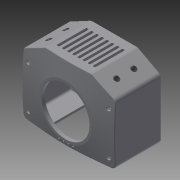
# Autodesk Inventor part: Enclosure01
Saved by Autodesk Inventor 2013 (Build 170138000, 138)
## iProperties
Created: 2014-04-13
Part Number: Enclosure01
Material: Generic
Document SubType Name: Modeling
Designer: spichelh
Density: 1 g/cm^3
Author: spichelh
Autodesk Inventor part; units mm, degrees
ref_plane "YZ Plane" through (0, 0, 0) normal (1, 0, 0) x (0, 1, 0)
ref_plane "XZ Plane" through (0, 0, 0) normal (0, 1, 0) x (-1, 0, 0)
ref_plane "XY Plane" through (0, 0, 0) normal (0, 0, 1) x (1, 0, 0)
sketch "Sketch1" plane through (0, 0, 0) normal (0, 0, 1) x (1, 0, 0)
  circle A0 centre (31.4469, 31.0185) radius 28
  line L0 (-19.3531, 19.423) -> (82.2469, 19.423) construction
  line L1 (7.9639, 76.573) -> (-19.3531, 76.573) construction
  line L2 (82.2469, 76.573) -> (53.8439, 76.573) construction
  line L3 (82.2469, 19.423) -> (82.2469, 76.573) construction
  line L4 (-19.3531, 76.573) -> (-19.3531, 19.423) construction
  line L5 (5.509, 60.2207) -> (61.389, 60.2207) construction
  line L6 (61.389, 60.2207) -> (61.389, 72.2207) construction
  line L7 (61.389, 72.2207) -> (5.509, 72.2207) construction
  line L8 (5.509, 72.2207) -> (5.509, 60.2207) construction
  circle A1 centre (61.389, 6.2635) radius 1.5 construction
  circle A2 centre (61.389, 55.7935) radius 1.5 construction
  circle A3 centre (5.509, 55.7935) radius 1.5 construction
  circle A4 centre (5.0259, 23.233) radius 1.5 construction
  arc A5 (5.509, 7.6907) -> (5.509, 1.6907) centre (5.509, 4.6907) ccw construction
  line L9 (5.509, 1.6907) -> (5.509, -3.7465) construction
  line L10 (5.509, -3.7465) -> (61.389, -3.7465) construction
  line L11 (61.389, -3.7465) -> (61.389, 1.6907) construction
  arc A6 (61.389, 1.6907) -> (61.389, 7.6907) centre (61.389, 4.6907) ccw construction
  line L12 (61.389, 7.6907) -> (61.389, 51.2207) construction
  arc A7 (61.389, 51.2207) -> (61.389, 57.2207) centre (61.389, 54.2207) ccw construction
  line L13 (61.389, 57.2207) -> (61.389, 60.2207) construction
  line L14 (61.389, 60.2207) -> (5.509, 60.2207) construction
  line L15 (5.509, 60.2207) -> (5.509, 57.2207) construction
  arc A8 (5.509, 57.2207) -> (5.509, 51.2207) centre (5.509, 54.2207) ccw construction
  line L16 (5.509, 51.2207) -> (5.509, 7.6907) construction
  line L17 (-22.3531, -3.7465) -> (85.2469, -3.7465)
  line L18 (85.2469, -3.7465) -> (85.2469, 66.2535)
  line L19 (58.3159, 80.573) -> (4.578, 80.573)
  line L20 (31.4469, -3.7465) -> (31.4469, 78.2535) construction
  circle A9 centre (31.4469, 31.0185) radius 23 projected
  line L21 (-22.3531, 66.2535) -> (4.578, 80.573)
  line L22 (-22.3531, 66.2535) -> (-22.3531, -3.7465)
  line L23 (85.2469, 66.2535) -> (58.3159, 80.573)
  point P0 (0, 0)
  dimension "d42" = 0
  dimension "d44" = 3
  dimension "d45" = 4
  dimension "d46" = 4
  dimension "d47" = 57.15
  dimension "d48" = 57.15
  dimension "d49" = 101.6
  dimension "d50" = 3.81
  dimension "d59" = 56
  dimension "d199" = 70
  dimension "d200" = 118
  dimension "d201" = 84.3195
  dimension "d202" = 107.6
  constraints: 48 end point, 9 centre point, 8 point on circle, 2 parallel, 2 symmetric about line, 1 concentric, 1 horizontal, 1 midpoint, 1 perpendicular, 1 point on line
  measures "d42" distance between parallel lines of L17 L10
  measures "d44" distance between parallel lines of L18 L3
  measures "d45" distance between parallel lines of L19 L1
  measures "d46" distance between parallel lines of L19 L2
  measures "d47" distance between parallel lines of L0 L1
  measures "d48" distance between parallel lines of L2 L0
  measures "d49" distance between parallel lines of L4 L3
  measures "d50" distance from line of L0 A4.centre
  measures "d59" diameter of A0
  measures "d199" distance of L21.start L17.start
  measures "d200" angle of L22 L21
  measures "d201" distance between parallel lines of L17 L19
  measures "d202" distance between parallel lines of L22 L18
extrude "Extrusion1" add sketch "Sketch1" along normal blind 11 contours L22 L21 L19 L23 L18 L17
sketch "Sketch4" plane through (0, 0, 11) normal (0, 0, 1) x (1, 0, 0)
  circle A0 centre (-15.5431, 55.7835) radius 1.5 projected
  circle A1 centre (-15.5431, 6.2535) radius 1.5 projected
  circle A2 centre (78.4369, 6.2535) radius 1.5 projected
  circle A3 centre (78.4369, 55.7835) radius 1.5 projected
  point P0 (0, 0)
extrude "Extrusion3" cut sketch "Sketch4" against normal blind 10
sketch "Sketch25" plane through (0, 0, 11) normal (0, 0, 1) x (1, 0, 0)
  circle A0 centre (31.4469, 31.019) radius 31
  circle A1 centre (31.4469, 31.019) radius 28
  line L0 (58.3159, 80.573) -> (4.578, 80.573) projected
  circle A2 centre (31.4469, 31.0185) radius 28 projected
  point P0 (0, 0)
  dimension "d196" = 62
  dimension "d198" = 49.554
  dimension "d203" = 0.0005
  constraints: 2 centre point, 1 coincident
  measures "d196" diameter of A0
  measures "d198" distance from line of L0 A0.centre
  measures "d203" distance of A0.centre A2.centre
extrude "Extrusion21" cut sketch "Sketch25" against normal blind 50 draft 82 contours A0 | A1 keep common part
sketch "Sketch2" plane through (0, 0, 0) normal (0, 0, -1) x (-1, 0, 0)
  circle A0 centre (-31.4469, 31.0185) radius 28 projected
  line L0 (22.3531, -3.7465) -> (-85.2469, -3.7465) projected
  line L1 (-58.3159, 80.573) -> (-4.578, 80.573) projected
  line L2 (-85.2469, -3.7465) -> (-85.2469, 66.2535) projected
  line L3 (-82.7469, 78.073) -> (19.8531, 78.073)
  line L4 (19.8531, 78.073) -> (19.8531, -1.2465)
  line L5 (19.8531, -1.2465) -> (-82.7469, -1.2465)
  line L6 (-82.7469, -1.2465) -> (-82.7469, 78.073)
  line L7 (22.3531, 66.2535) -> (22.3531, -3.7465) projected
  line L8 (-4.578, 80.573) -> (22.3531, 66.2535) projected
  line L9 (-85.2469, 66.2535) -> (-58.3159, 80.573) projected
  dimension "d51" = 2.5
  dimension "d52" = 2.5
  dimension "d54" = 2.5
  constraints: 8 end point, 2 parallel, 1 horizontal, 1 perpendicular
  measures "d51" distance between parallel lines of L3 L1
  measures "d52" distance between parallel lines of L2 L6
  measures "d54" distance between parallel lines of L0 L5
extrude "Extrusion2" add sketch "Sketch2" along normal blind 38 contours L0 L2 L9 L6 L5 L4 L8 L7 | L3 L9 L1 L8
ref_plane "Work Plane1" through (0, 0, 7) normal (0, 0, -1) x (-1, 0, 0)
sketch "Sketch28" plane through (0, 0, 7) normal (0, 0, -1) x (-1, 0, 0)
  circle A0 centre (-31.4469, 31.0185) radius 28 projected
  circle A1 centre (-31.4469, 31.0185) radius 31
  point P0 (0, 0)
  dimension "d209" = 62
  constraints: 1 centre point, 1 coincident
  measures "d209" diameter of A1
extrude "Extrusion23" cut sketch "Sketch28" along normal blind 50 draft 78 contours A0 | A1
sketch "Sketch5" plane through (-22.3531, 80.573, 10) normal (0, 1, 0) x (-1, 0, 0)
  line L0 (0, 0) -> (128.1647, 0)
  line L1 (36.0824, 63) -> (92.0824, 63)
  line L2 (92.0824, 63) -> (92.0824, 7)
  line L3 (92.0824, 7) -> (36.0824, 7)
  line L4 (36.0824, 7) -> (36.0824, 63)
  line L5 (64.0824, 0) -> (64.0824, -31.7336) construction
  line L6 (36.0824, 63) -> (92.0824, 7) construction
  line L7 (92.0824, 63) -> (36.0824, 7) construction
  line L8 (104.9242, 0) -> (-0.6758, 0)
  line L9 (87.1496, -1) -> (20.4504, -1) projected
  line L10 (-26.931, -48) -> (-80.669, -48) projected
  line L11 (16.7879, -48) -> (43.5691, -1) construction
  point P0 (19.351, -30)
  point P1 (64.0824, 35)
  point P2 (0, 48)
  point P3 (64.0824, 35)
  point P4 (20.4504, -1)
  dimension "d28" = 56
  dimension "d29" = 56
  dimension "d41" = 7
  constraints: 20 end point, 3 midpoint, 3 parallel, 2 point on line, 1 collinear, 1 horizontal, 1 perpendicular, 4 other
  measures "d28" distance of L2.end L3.end
  measures "d29" distance of L1.end L2.end
  measures "d41" distance between parallel lines of L8 L3
extrude "Extrusion4" cut sketch "Sketch5" against normal blind 100
sketch "Sketch6" plane through (-6.7798, 80.573, 3) normal (0, 1, 0) x (1, 0, 0)
  line L0 (71.5763, -7) -> (-25.8, -7) projected
  line L1 (0, 0) -> (56, 0)
  line L2 (56, 0) -> (56, -7)
  line L3 (56, -7) -> (0, -7)
  line L4 (0, -7) -> (0, 0)
  point P0 (76.8, -7)
  point P1 (-20.8, -7)
  point P2 (6.7798, 3)
  point P3 (71.5763, -8)
  point P4 (-25.8, -7)
  constraints: 8 end point, 2 parallel, 1 horizontal, 1 perpendicular, 2 other
extrude "Extrusion5" [suppressed]
fillet "Fillet9" radius 5 6 edges at (85.2469, -3.7465, 3.1642) (-22.3531, -3.7465, 3.1642) (-22.3531, 66.2535, 3.1189) (4.578, 80.573, 4.521) (58.3159, 80.573, 4.521) (85.2469, 66.2535, 3.1189)
sketch "Sketch24" plane through (31.4469, 31.0185, 3) normal (0, 0, -1) x (0.9394635, -0.3426491, 0)
  arc A0 (-28, 0) -> (28, 0) centre (0, 0) ccw projected
  circle A1 centre (0, 0) radius 28
  point P0 (-18.9148, 39.916)
  dimension "d186" = 56
  constraints: 1 centre point, 1 coincident
  measures "d186" diameter of A1
extrude "Extrusion20" [suppressed]
ref_plane "Work Plane2" through (0, 0, 6) normal (0, 0, 1) x (1, 0, 0)
sketch "Sketch7" plane through (0, 0, 11) normal (0, 0, 1) x (1, 0, 0)
  line L0 (-22.3531, -3.7465) -> (85.2469, -3.7465) projected
  line L1 (59.4469, 75.7535) -> (3.4469, 75.7535) projected
  line L2 (31.4469, -3.7465) -> (31.4469, 75.7535) construction
  line L3 (23.1969, -0.7465) -> (23.1969, -0.7465)
  line L4 (22.1969, 0.2535) -> (22.1969, 1.2535)
  line L5 (23.1969, 2.2535) -> (23.1969, 2.2535)
  line L6 (24.1969, 1.2535) -> (24.1969, 0.2535)
  arc A0 (24.1969, 1.2535) -> (23.1969, 2.2535) centre (23.1969, 1.2535) ccw
  arc A1 (23.1969, 2.2535) -> (22.1969, 1.2535) centre (23.1969, 1.2535) ccw
  arc A2 (22.1969, 0.2535) -> (23.1969, -0.7465) centre (23.1969, 0.2535) ccw
  arc A3 (23.1969, -0.7465) -> (24.1969, 0.2535) centre (23.1969, 0.2535) ccw
  line L7 (27.6969, 0.2535) -> (27.6969, 1.2535)
  line L8 (29.6969, 1.2535) -> (29.6969, 0.2535)
  arc A4 (29.6969, 1.2535) -> (28.6969, 2.2535) centre (28.6969, 1.2535) ccw
  arc A5 (28.6969, 2.2535) -> (27.6969, 1.2535) centre (28.6969, 1.2535) ccw
  arc A6 (27.6969, 0.2535) -> (28.6969, -0.7465) centre (28.6969, 0.2535) ccw
  arc A7 (28.6969, -0.7465) -> (29.6969, 0.2535) centre (28.6969, 0.2535) ccw
  line L9 (33.1969, 0.2535) -> (33.1969, 1.2535)
  line L10 (35.1969, 1.2535) -> (35.1969, 0.2535)
  arc A8 (35.1969, 1.2535) -> (34.1969, 2.2535) centre (34.1969, 1.2535) ccw
  arc A9 (34.1969, 2.2535) -> (33.1969, 1.2535) centre (34.1969, 1.2535) ccw
  arc A10 (33.1969, 0.2535) -> (34.1969, -0.7465) centre (34.1969, 0.2535) ccw
  arc A11 (34.1969, -0.7465) -> (35.1969, 0.2535) centre (34.1969, 0.2535) ccw
  line L11 (38.6969, 0.2535) -> (38.6969, 1.2535)
  line L12 (40.6969, 1.2535) -> (40.6969, 0.2535)
  arc A12 (40.6969, 1.2535) -> (39.6969, 2.2535) centre (39.6969, 1.2535) ccw
  arc A13 (39.6969, 2.2535) -> (38.6969, 1.2535) centre (39.6969, 1.2535) ccw
  arc A14 (38.6969, 0.2535) -> (39.6969, -0.7465) centre (39.6969, 0.2535) ccw
  arc A15 (39.6969, -0.7465) -> (40.6969, 0.2535) centre (39.6969, 0.2535) ccw
  line L13 (29.6969, 0.7535) -> (33.1969, 0.7535) construction
  point P0 (-17.3531, -3.7465)
  point P1 (80.2469, -3.7465)
  point P2 (0, 0)
  point P3 (24.1969, -0.7465)
  point P4 (22.1969, 2.2535)
  point P5 (24.1969, 2.2535)
  point P6 (29.6969, -0.7465)
  point P7 (27.6969, 2.2535)
  point P8 (29.6969, 2.2535)
  point P9 (35.1969, -0.7465)
  point P10 (33.1969, 2.2535)
  point P11 (35.1969, 2.2535)
  point P12 (40.6969, -0.7465)
  point P13 (38.6969, 2.2535)
  point P14 (40.6969, 2.2535)
  point P15 (31.4469, 0.7535)
  dimension "d64" = 2
  dimension "d66" = 3
  dimension "d67" = 1
  dimension "d68" = 1
  dimension "d69" = 4
  dimension "d78" = 16.5
  dimension "d79" = 7.25
  dimension "d80" = 7.25
  constraints: 32 point on circle, 24 end point, 16 centre point, 16 point on line, 8 tangent, 5 midpoint, 2 equal radius, 2 parallel, 1 horizontal, 1 perpendicular
  measures "d64" distance of point (22.197, 2.253) point (24.197, 2.253)
  measures "d66" distance of point (24.197, 2.253) point (24.197, -0.747)
  measures "d67" radius of A0
  measures "d68" radius of A3
  measures "d69" distance from line of L0 A3.centre
  measures "d78" distance of A14.centre A3.centre
  measures "d79" distance from line of L6 point (31.447, 0.753)
  measures "d80" distance from line of point (31.447, 0.753) L11
extrude "Extrusion6" cut sketch "Sketch7" against normal blind 5
sketch "Sketch31" plane through (0, 0, 6) normal (0, 0, 1) x (1, 0, 0)
  line L0 (85.2469, 1.2535) -> (85.2469, 63.2492) projected
  line L1 (82.5943, 67.6639) -> (59.4166, 79.9877) projected
  line L2 (57.0693, 80.573) -> (5.8246, 80.573) projected
  line L3 (3.4773, 79.9877) -> (-19.7004, 67.6639) projected
  line L4 (-22.3531, 63.2492) -> (-22.3531, 1.2535) projected
  line L5 (-17.3531, -3.7465) -> (80.2469, -3.7465) projected
  arc A0 (29.6799, 0.0694) -> (33.214, 0.0694) centre (31.4469, 31.019) ccw projected
  arc A1 (24.1969, 0.8787) -> (27.697, 0.2466) centre (31.4469, 31.019) ccw projected
  line L6 (24.1969, 0.8787) -> (24.1969, 0.2535) projected
  line L7 (22.1969, 0.2535) -> (22.1969, 1.2535) projected
  arc A2 (40.6819, 1.4265) -> (22.212, 1.4265) centre (31.4469, 31.019) ccw projected
  line L8 (40.6969, 1.2535) -> (40.6969, 0.2535) projected
  line L9 (38.6969, 0.2535) -> (38.6969, 0.8787) projected
  arc A3 (35.1969, 0.2466) -> (38.6969, 0.8787) centre (31.4469, 31.019) ccw projected
  spline S0 degree 5 poles (79.9369, 6.2535) (79.9369, 6.4896) (79.8901, 6.7131) (79.8078, 6.9142) (79.6985, 7.089) (79.3892, 7.444) (79.1712, 7.6007) (78.9248, 7.7086) (78.6593, 7.7625) (78.197, 7.7457) (78.0071, 7.7107) (77.815, 7.6419) (77.6284, 7.5361) (77.2941, 7.2495) (77.1462, 7.0707) (77.0327, 6.8552) (76.9691, 6.6321) (76.9219, 6.1944) (76.9403, 5.9806) (76.9923, 5.7833) (77.0708, 5.6069) (77.3344, 5.1912) (77.5564, 4.9876) (77.8147, 4.8424) (78.1045, 4.759) (78.6051, 4.7503) (78.8055, 4.7777) (79.0097, 4.8419) (79.2089, 4.9467) (79.5873, 5.2569) (79.7624, 5.4705) (79.8851, 5.7352) (79.9369, 6.0009) (79.9369, 6.2535) knots 0 0 0 0 0 0 0.115502 0.115502 0.115502 0.115502 0.273569 0.273569 0.273569 0.273569 0.379516 0.379516 0.379516 0.379516 0.484537 0.484537 0.484537 0.484537 0.590505 0.590505 0.590505 0.590505 0.765499 0.765499 0.765499 0.765499 0.876442 0.876442 0.876442 0.876442 1 1 1 1 1 1 projected
  spline S1 degree 5 poles (-14.0431, 55.7835) (-14.0431, 56.0034) (-14.0836, 56.2117) (-14.1553, 56.401) (-14.2511, 56.5681) (-14.5342, 56.9259) (-14.7425, 57.0919) (-14.9815, 57.2113) (-15.2422, 57.2785) (-15.7112, 57.2866) (-15.9117, 57.2593) (-16.1159, 57.1951) (-16.3151, 57.0902) (-16.6735, 56.7964) (-16.8328, 56.6087) (-16.9533, 56.3798) (-17.0179, 56.1423) (-17.0573, 55.6805) (-17.031, 55.457) (-16.9684, 55.2523) (-16.8776, 55.0716) (-16.5871, 54.6638) (-16.3545, 54.472) (-16.0886, 54.3411) (-15.7951, 54.2733) (-15.3031, 54.2912) (-15.1133, 54.3263) (-14.9212, 54.3951) (-14.7345, 54.5009) (-14.3755, 54.8087) (-14.208, 55.0203) (-14.0917, 55.2804) (-14.0431, 55.5385) (-14.0431, 55.7835) knots 0 0 0 0 0 0 0.108338 0.108338 0.108338 0.108338 0.265313 0.265313 0.265313 0.265313 0.376257 0.376257 0.376257 0.376257 0.487434 0.487434 0.487434 0.487434 0.598396 0.598396 0.598396 0.598396 0.773389 0.773389 0.773389 0.773389 0.879335 0.879335 0.879335 0.879335 1 1 1 1 1 1 projected
  spline S2 degree 5 poles (-14.0431, 6.2535) (-14.0431, 6.4984) (-14.0918, 6.7565) (-14.208, 7.0166) (-14.3755, 7.2282) (-14.7345, 7.5361) (-14.9212, 7.6419) (-15.1133, 7.7107) (-15.3031, 7.7457) (-15.7951, 7.7636) (-16.0886, 7.6958) (-16.3545, 7.5649) (-16.5871, 7.3732) (-16.8776, 6.9654) (-16.9684, 6.7847) (-17.031, 6.58) (-17.0573, 6.3564) (-17.0179, 5.8947) (-16.9533, 5.6571) (-16.8328, 5.4282) (-16.6735, 5.2406) (-16.3151, 4.9467) (-16.1159, 4.8419) (-15.9117, 4.7777) (-15.7112, 4.7503) (-15.2403, 4.7585) (-14.9778, 4.8266) (-14.7375, 4.9476) (-14.5284, 5.1157) (-14.2473, 5.4757) (-14.1531, 5.6418) (-14.0828, 5.8295) (-14.0431, 6.0358) (-14.0431, 6.2535) knots 0 0 0 0 0 0 0.120665 0.120665 0.120665 0.120665 0.226611 0.226611 0.226611 0.226611 0.401603 0.401603 0.401603 0.401603 0.512565 0.512565 0.512565 0.512565 0.623742 0.623742 0.623742 0.623742 0.734686 0.734686 0.734686 0.734686 0.892762 0.892762 0.892762 0.892762 1 1 1 1 1 1 projected
  spline S3 degree 5 poles (79.9369, 55.7835) (79.9369, 56.036) (79.885, 56.3017) (79.7624, 56.5664) (79.5873, 56.78) (79.2089, 57.0902) (79.0097, 57.1951) (78.8055, 57.2593) (78.6051, 57.2866) (78.1045, 57.2779) (77.8147, 57.1946) (77.5564, 57.0494) (77.3344, 56.8457) (77.0708, 56.43) (76.9923, 56.2537) (76.9403, 56.0564) (76.9219, 55.8426) (76.9691, 55.4049) (77.0327, 55.1817) (77.1462, 54.9663) (77.2941, 54.7875) (77.6284, 54.5009) (77.815, 54.3951) (78.0071, 54.3263) (78.197, 54.2912) (78.6612, 54.2743) (78.9285, 54.3291) (79.1763, 54.4385) (79.3953, 54.5974) (79.7026, 54.9547) (79.8101, 55.1285) (79.891, 55.3281) (79.9369, 55.5496) (79.9369, 55.7835) knots 0 0 0 0 0 0 0.123558 0.123558 0.123558 0.123558 0.234501 0.234501 0.234501 0.234501 0.409495 0.409495 0.409495 0.409495 0.515462 0.515462 0.515462 0.515462 0.620483 0.620483 0.620483 0.620483 0.726431 0.726431 0.726431 0.726431 0.885598 0.885598 0.885598 0.885598 1 1 1 1 1 1 projected
  line L10 (-14.4969, 56.8585) -> (-16.5892, 54.7085) construction
  line L11 (-16.618, 56.8296) -> (-14.4681, 54.7373) construction
  circle A4 centre (-15.5431, 55.7835) radius 2.5
  line L12 (31.4469, 31.019) -> (31.4469, 90.1404) construction
  circle A5 centre (78.4369, 55.7835) radius 2.5
  line L13 (31.4469, 31.019) -> (51.7757, 31.019) construction
  circle A6 centre (-15.5431, 6.2545) radius 2.5
  circle A7 centre (78.4369, 6.2545) radius 2.5
  point P0 (0, 0)
  dimension "d214" = 5
  constraints: 8 end point, 4 centre point, 3 symmetric about line, 2 horizontal alignment, 2 midpoint, 2 perpendicular, 1 coincident, 1 parallel, 25 other
  measures "d214" diameter of A4
extrude "Extrusion24" cut sketch "Sketch31" along normal blind 6
fillet "Fillet11" radius 1 13 edges at (-21.651, 65.8041, 6.4356) (-22.3531, 32.0868, 7.7942) (-20.7245, -2.4389, 6.6463) (31.4469, -3.7465, 10.4708) (83.6183, -2.4389, 6.6463) (85.2469, 46.5053, 7.4887) (85.2469, 16.6408, 7.5303) (84.5449, 65.8041, 6.4356) (70.6846, 73.9964, 7.178) (58.2489, 80.4318, 7.4565) (31.4469, 80.573, 8.3924) (4.6451, 80.4318, 7.4565) (-7.7907, 73.9964, 7.178)
ref_plane "Work Plane3" through (0, 0, 4) normal (0, 0, -1) x (-1, 0, 0)
sketch "Sketch33" plane through (0, 0, 4) normal (0, 0, -1) x (-1, 0, 0)
  arc A0 (-38.6969, 0.8782) -> (-35.1969, 0.2461) centre (-31.4469, 31.0185) ccw projected
  line L0 (-38.6969, 0.8782) -> (-38.6969, 0.2535) projected
  line L1 (-40.6969, 0.2535) -> (-40.6969, 1.2535) projected
  arc A1 (-22.2119, 1.426) -> (-40.6819, 1.426) centre (-31.4469, 31.0185) ccw projected
  line L2 (-22.1969, 1.2535) -> (-22.1969, 0.2535) projected
  line L3 (-24.1969, 0.2535) -> (-24.1969, 0.8782) projected
  arc A2 (-27.697, 0.2461) -> (-24.1969, 0.8782) centre (-31.4469, 31.0185) ccw projected
  arc A3 (-33.2141, 0.0689) -> (-29.6798, 0.0689) centre (-31.4469, 31.0185) ccw projected
  spline S0 degree 5 poles (-85.2469, 63.2492) (-85.2469, 63.4652) (-85.2353, 63.6853) (-85.2111, 63.9087) (-85.1734, 64.1344) (-85.0962, 64.4729) (-85.0672, 64.5853) (-85.0347, 64.6976) (-84.9987, 64.8097) (-84.9339, 64.9922) (-84.9073, 65.0629) (-84.8793, 65.1334) (-84.8498, 65.2035) (-84.7518, 65.425) (-84.6779, 65.5749) (-84.5974, 65.7222) (-84.5106, 65.8663) (-84.2952, 66.1922) (-84.162, 66.3712) (-84.0195, 66.5417) (-83.8691, 66.7028) (-83.6384, 66.9246) (-83.5633, 66.9931) (-83.4869, 67.0594) (-83.4094, 67.1233) (-83.1887, 67.2962) (-83.0433, 67.3998) (-82.8953, 67.4956) (-82.7455, 67.5835) (-82.5943, 67.6639) knots 0 0 0 0 0 0 0.217399 0.217399 0.217399 0.217399 0.325184 0.325184 0.325184 0.325184 0.393663 0.393663 0.393663 0.393663 0.542664 0.542664 0.542664 0.542664 0.740085 0.740085 0.740085 0.740085 0.832658 0.832658 0.832658 0.832658 1 1 1 1 1 1 projected
  line L4 (-85.2469, 1.2535) -> (-85.2469, 63.2492) projected
  spline S1 degree 6 poles (-80.2469, -3.7465) (-80.6265, -3.7465) (-81.0155, -3.712) (-81.4128, -3.6396) (-81.8151, -3.525) (-82.2171, -3.3637) (-82.7463, -3.0797) (-82.8803, -3.0014) (-83.0129, -2.9172) (-83.1438, -2.8269) (-83.2726, -2.7305) (-83.4692, -2.5708) (-83.5389, -2.5117) (-83.6076, -2.4507) (-83.6754, -2.3879) (-83.742, -2.3232) (-83.9403, -2.1222) (-84.0681, -1.9803) (-84.1903, -1.8315) (-84.3059, -1.6765) (-84.4145, -1.5159) (-84.5868, -1.2333) (-84.6545, -1.1137) (-84.7182, -0.992) (-84.7776, -0.8686) (-84.8327, -0.7438) (-84.9063, -0.5615) (-84.9282, -0.5048) (-84.9493, -0.448) (-84.9694, -0.391) (-84.9887, -0.3338) (-85.0364, -0.1852) (-85.0636, -0.0936) (-85.0885, -0.0019) (-85.1111, 0.0899) (-85.1316, 0.1816) (-85.1831, 0.4393) (-85.2092, 0.605) (-85.2284, 0.7696) (-85.2409, 0.9328) (-85.2469, 1.0942) (-85.2469, 1.2535) knots 0 0 0 0 0 0 0 0.347573 0.347573 0.347573 0.347573 0.347573 0.466572 0.466572 0.466572 0.466572 0.466572 0.533142 0.533142 0.533142 0.533142 0.533142 0.668156 0.668156 0.668156 0.668156 0.668156 0.763955 0.763955 0.763955 0.763955 0.763955 0.80693 0.80693 0.80693 0.80693 0.80693 0.875527 0.875527 0.875527 0.875527 0.875527 1 1 1 1 1 1 1 projected
  line L5 (17.3531, -3.7465) -> (-80.2469, -3.7465) projected
  spline S2 degree 6 poles (22.3531, 1.2535) (22.3531, 1.0855) (22.3463, 0.9153) (22.3324, 0.7431) (22.3111, 0.5692) (22.282, 0.3944) (22.2266, 0.1327) (22.2064, 0.0462) (22.1843, -0.0403) (22.1601, -0.1268) (22.134, -0.2131) (22.0472, -0.4788) (21.9798, -0.6575) (21.9037, -0.8343) (21.819, -1.0082) (21.7261, -1.1784) (21.5542, -1.4612) (21.4789, -1.5763) (21.4, -1.6886) (21.3176, -1.7981) (21.232, -1.9044) (21.1038, -2.0534) (21.0635, -2.0989) (21.0227, -2.1437) (20.9813, -2.1877) (20.9394, -2.2311) (20.8312, -2.3398) (20.7642, -2.4041) (20.6962, -2.4666) (20.6271, -2.5273) (20.5571, -2.5861) (20.3598, -2.7448) (20.2306, -2.8406) (20.0992, -2.9303) (19.9662, -3.0139) (19.8318, -3.0915) (19.3055, -3.3708) (18.907, -3.529) (18.5084, -3.6415) (18.1147, -3.7126) (17.7292, -3.7465) (17.3531, -3.7465) knots 0 0 0 0 0 0 0 0.13123 0.13123 0.13123 0.13123 0.13123 0.195895 0.195895 0.195895 0.195895 0.195895 0.330929 0.330929 0.330929 0.330929 0.330929 0.42672 0.42672 0.42672 0.42672 0.42672 0.469685 0.469685 0.469685 0.469685 0.469685 0.536329 0.536329 0.536329 0.536329 0.536329 0.655502 0.655502 0.655502 0.655502 0.655502 1 1 1 1 1 1 1 projected
  line L6 (22.3531, 63.2492) -> (22.3531, 1.2535) projected
  spline S3 degree 5 poles (19.7004, 67.6639) (19.8516, 67.5835) (20.0014, 67.4956) (20.1494, 67.3998) (20.2948, 67.2962) (20.5155, 67.1233) (20.593, 67.0594) (20.6694, 66.9931) (20.7445, 66.9246) (20.9752, 66.7028) (21.1257, 66.5417) (21.2681, 66.3712) (21.4013, 66.1922) (21.6167, 65.8663) (21.7035, 65.7222) (21.784, 65.5749) (21.8579, 65.425) (21.9559, 65.2035) (21.9854, 65.1334) (22.0134, 65.0629) (22.04, 64.9922) (22.1048, 64.8097) (22.1408, 64.6976) (22.1733, 64.5853) (22.2024, 64.4729) (22.2796, 64.1344) (22.3172, 63.9087) (22.3414, 63.6853) (22.3531, 63.4652) (22.3531, 63.2492) knots 0 0 0 0 0 0 0.167342 0.167342 0.167342 0.167342 0.259915 0.259915 0.259915 0.259915 0.457336 0.457336 0.457336 0.457336 0.606337 0.606337 0.606337 0.606337 0.674816 0.674816 0.674816 0.674816 0.782601 0.782601 0.782601 0.782601 1 1 1 1 1 1 projected
  line L7 (-3.4773, 79.9877) -> (19.7004, 67.6639) projected
  spline S4 degree 6 poles (-5.8246, 80.573) (-5.6769, 80.573) (-5.5274, 80.5677) (-5.3764, 80.557) (-5.2242, 80.5406) (-5.0711, 80.5183) (-4.674, 80.4451) (-4.4291, 80.3849) (-4.1849, 80.309) (-3.9434, 80.2172) (-3.7067, 80.1097) (-3.4773, 79.9877) knots 0 0 0 0 0 0 0 0.38665 0.38665 0.38665 0.38665 0.38665 1 1 1 1 1 1 1 projected
  line L8 (-57.0693, 80.573) -> (-5.8246, 80.573) projected
  spline S5 degree 6 poles (-59.4166, 79.9877) (-59.195, 80.1055) (-58.9667, 80.2098) (-58.7337, 80.2996) (-58.4981, 80.3744) (-58.2617, 80.4346) (-57.8643, 80.5121) (-57.7027, 80.537) (-57.5421, 80.5552) (-57.3827, 80.5671) (-57.225, 80.573) (-57.0693, 80.573) knots 0 0 0 0 0 0 0 0.592396 0.592396 0.592396 0.592396 0.592396 1 1 1 1 1 1 1 projected
  line L9 (-82.5943, 67.6639) -> (-59.4166, 79.9877) projected
  line L10 (-82.7469, 1.2535) -> (-82.7469, 63.2492)
  line L11 (-81.4206, 65.4565) -> (-58.2429, 77.7803)
  line L12 (-57.0693, 78.073) -> (-5.8246, 78.073)
  line L13 (-4.651, 77.7803) -> (18.5267, 65.4565)
  line L14 (19.8531, 63.2492) -> (19.8531, 1.2535)
  line L15 (17.3531, -1.2465) -> (-80.2469, -1.2465)
  spline S6 degree 5 poles (-80.2469, -1.2465) (-81.0321, -1.2463) (-81.8186, -0.9392) (-82.4396, -0.3182) (-82.7467, 0.4683) (-82.7469, 1.2535) knots 0 0 0 0 0 0 1 1 1 1 1 1
  spline S7 degree 4 poles (-82.7469, 63.2492) (-82.7472, 63.9249) (-82.5019, 64.6041) (-82.0174, 65.1395) (-81.4206, 65.4565) knots 0 0 0 0 0 1 1 1 1 1
  spline S8 degree 3 poles (-58.2429, 77.7803) (-57.8835, 77.9719) (-57.4766, 78.0734) (-57.0693, 78.073) knots 0 0 0 0 1 1 1 1
  spline S9 degree 3 poles (-5.8246, 78.073) (-5.4173, 78.0734) (-5.0104, 77.9719) (-4.651, 77.7803) knots 0 0 0 0 1 1 1 1
  spline S10 degree 4 poles (18.5267, 65.4565) (19.1235, 65.1395) (19.608, 64.6041) (19.8533, 63.9249) (19.8531, 63.2492) knots 0 0 0 0 0 1 1 1 1 1
  spline S11 degree 5 poles (19.8531, 1.2535) (19.8528, 0.4683) (19.5457, -0.3182) (18.9247, -0.9392) (18.1383, -1.2463) (17.3531, -1.2465) knots 0 0 0 0 0 0 1 1 1 1 1 1
  point P0 (0, 0)
  dimension "d223" = 2.5
  constraints: 12 end point, 11 parallel, 2 horizontal alignment, 32 other
  measures "d223" distance between parallel lines of L5 L15
extrude "Extrusion26" add sketch "Sketch33" along normal blind 50
sketch "Sketch34" plane through (5.8246, 80.573, -46) normal (0, 1, 0) x (1, 0, 0)
  line L0 (0, -47.7314) -> (0, 0) projected
  line L1 (4, -45) -> (5, -45)
  line L2 (6, -44) -> (6, -11)
  line L3 (5, -10) -> (4, -10)
  line L4 (3, -11) -> (3, -44)
  arc A0 (6, -11) -> (5, -10) centre (5, -11) ccw
  arc A1 (4, -10) -> (3, -11) centre (4, -11) ccw
  arc A2 (3, -44) -> (4, -45) centre (4, -44) ccw
  arc A3 (5, -45) -> (6, -44) centre (5, -44) ccw
  line L5 (56.6223, -57) -> (-5.3777, -57) projected
  line L6 (10, -45) -> (11, -45)
  line L7 (12, -44) -> (12, -11)
  line L8 (11, -10) -> (10, -10)
  line L9 (9, -11) -> (9, -44)
  arc A4 (12, -11) -> (11, -10) centre (11, -11) ccw
  arc A5 (10, -10) -> (9, -11) centre (10, -11) ccw
  arc A6 (9, -44) -> (10, -45) centre (10, -44) ccw
  arc A7 (11, -45) -> (12, -44) centre (11, -44) ccw
  line L10 (16, -45) -> (17, -45)
  line L11 (18, -44) -> (18, -11)
  line L12 (17, -10) -> (16, -10)
  line L13 (15, -11) -> (15, -44)
  arc A8 (18, -11) -> (17, -10) centre (17, -11) ccw
  arc A9 (16, -10) -> (15, -11) centre (16, -11) ccw
  arc A10 (15, -44) -> (16, -45) centre (16, -44) ccw
  arc A11 (17, -45) -> (18, -44) centre (17, -44) ccw
  line L14 (22, -45) -> (23, -45)
  line L15 (24, -44) -> (24, -11)
  line L16 (23, -10) -> (22, -10)
  line L17 (21, -11) -> (21, -44)
  arc A12 (24, -11) -> (23, -10) centre (23, -11) ccw
  arc A13 (22, -10) -> (21, -11) centre (22, -11) ccw
  arc A14 (21, -44) -> (22, -45) centre (22, -44) ccw
  arc A15 (23, -45) -> (24, -44) centre (23, -44) ccw
  line L18 (28, -45) -> (29, -45)
  line L19 (30, -44) -> (30, -11)
  line L20 (29, -10) -> (28, -10)
  line L21 (27, -11) -> (27, -44)
  arc A16 (30, -11) -> (29, -10) centre (29, -11) ccw
  arc A17 (28, -10) -> (27, -11) centre (28, -11) ccw
  arc A18 (27, -44) -> (28, -45) centre (28, -44) ccw
  arc A19 (29, -45) -> (30, -44) centre (29, -44) ccw
  line L22 (34, -45) -> (35, -45)
  line L23 (36, -44) -> (36, -11)
  line L24 (35, -10) -> (34, -10)
  line L25 (33, -11) -> (33, -44)
  arc A20 (36, -11) -> (35, -10) centre (35, -11) ccw
  arc A21 (34, -10) -> (33, -11) centre (34, -11) ccw
  arc A22 (33, -44) -> (34, -45) centre (34, -44) ccw
  arc A23 (35, -45) -> (36, -44) centre (35, -44) ccw
  line L26 (40, -45) -> (41, -45)
  line L27 (42, -44) -> (42, -11)
  line L28 (41, -10) -> (40, -10)
  line L29 (39, -11) -> (39, -44)
  arc A24 (42, -11) -> (41, -10) centre (41, -11) ccw
  arc A25 (40, -10) -> (39, -11) centre (40, -11) ccw
  arc A26 (39, -44) -> (40, -45) centre (40, -44) ccw
  arc A27 (41, -45) -> (42, -44) centre (41, -44) ccw
  line L30 (46, -45) -> (47, -45)
  line L31 (48, -44) -> (48, -11)
  line L32 (47, -10) -> (46, -10)
  line L33 (45, -11) -> (45, -44)
  arc A28 (48, -11) -> (47, -10) centre (47, -11) ccw
  arc A29 (46, -10) -> (45, -11) centre (46, -11) ccw
  arc A30 (45, -44) -> (46, -45) centre (46, -44) ccw
  arc A31 (47, -45) -> (48, -44) centre (47, -44) ccw
  point P0 (-5.8246, -46)
  point P1 (16.3874, -57)
  point P2 (34.8572, -57)
  dimension "d226" = 3
  dimension "d228" = 35
  dimension "d229" = 1
  dimension "d230" = 12
  dimension "d231" = 3
  dimension "d234" = 6
  constraints: 64 end point, 64 point on circle, 32 centre point, 8 tangent, 3 equal radius, 2 horizontal, 2 parallel, 1 collinear, 1 perpendicular, 139 other
  measures "d226" distance between parallel lines of L4 L2
  measures "d228" distance between parallel lines of L3 L1
  measures "d229" radius of A0
  measures "d230" distance between parallel lines of L5 L1
  measures "d231" distance between parallel lines of L0 L4
  measures "d234" distance of L2.start L7.start
extrude "Extrusion27" cut sketch "Sketch34" against normal blind 50
sketch "Sketch35" plane through (59.4166, 79.9877, 1.6023) normal (0.4694716, 0.8829476, 0) x (0.8829476, -0.4694716, 0)
  line L0 (26.2504, 1.3872) -> (26.2504, 47.6023) projected
  line L1 (0, 0) -> (0, 47.6023) projected
  line L2 (0, 10.6023) -> (26.2504, 10.6023) construction
  line L3 (29.2937, -9.3977) -> (-32.7063, -9.3977) construction
  point P0 (-14.9098, 1.6023)
  point P1 (4.0326, -9.3977)
  point P2 (20.3405, -9.3977)
  point P3 (13.1252, 10.6023)
  point P4 (13.1252, 30.6023)
  dimension "d241" = 20
  dimension "d244" = 20
  constraints: 2 end point, 2 point on line, 1 midpoint, 1 perpendicular, 1 vertical, 1 other
  measures "d241" distance between parallel lines of L3 L2
  measures "d244" distance of point (13.125, 10.602) point (13.125, 30.602)
hole "Hole3" at (71.0055, 73.8258, -9) at (71.0055, 73.8258, -29) direction (-0.4694716, -0.8829476, 0) diameter 6.35 depth 8 tip angle 118
sketch "Sketch36" plane through (58.2429, 77.7803, -46) normal (-0.4694716, -0.8829476, 0) x (0.8829476, -0.4694716, 0)
  circle A0 centre (13.1252, 37) radius 3.175 projected
  circle A1 centre (13.1252, 17) radius 3.175 projected
  circle A2 centre (13.1252, 17) radius 5.175
  circle A3 centre (13.1252, 37) radius 5.175
  point P0 (-14.9098, 46)
  dimension "d256" = 10.35
  dimension "d257" = 10.35
  constraints: 2 centre point, 2 coincident
  measures "d256" diameter of A2
  measures "d257" diameter of A3
extrude "Extrusion28" add sketch "Sketch36" along normal blind 5
sketch "Sketch37" plane through (67.4844, 67.2037, -29) normal (-0.4694716, -0.8829476, 0) x (0.8829476, -0.4694716, 0)
  circle A0 centre (0, 0) radius 5.175 projected
  circle A1 centre (0, 20) radius 3.175 projected
  circle A2 centre (0, 20) radius 5.175 projected
  point P0 (-28.035, 29)
extrude "Extrusion29" add sketch "Sketch37" along normal blind 2 contours A0 | A1 | A2
thread "Thread1" size "M7x1" class "6H" standard "ANSI Metric M Profile" full length
thread "Thread2" size "M7x1" class "6H" standard "ANSI Metric M Profile" full length
sketch "Sketch39" plane through (-17.3531, -1.2465, -46) normal (0, 1, 0) x (1, 0, 0)
  line L0 (80.3315, -50) -> (17.2685, -50) projected
  line L1 (97.6, -47.1543) -> (97.6, 0) projected
  line L2 (0, 0) -> (97.6, 0) projected
  line L3 (0, -47.1543) -> (0, 0) projected
  line L4 (97.6, -23.5771) -> (0, -23.5771) construction
  line L5 (48.8, -23.5771) -> (48.8, -5.5658) construction
  point P0 (17.3531, -46)
  constraints: 4 end point, 3 midpoint, 1 perpendicular, 2 other
ref_plane "Work Plane4" through (31.4469, -1.2465, -22.4229) normal (-1, 0, 0) x (0, 0, 1)
mirror "Mirror1" about plane through (31.4469, -1.2465, -22.4229) normal (-1, 0, 0) of "Hole3", "Extrusion28", "Extrusion29"
thread "Thread3" size "M7x1" class "6H" standard "ANSI Metric M Profile" full length
thread "Thread4" size "M7x1" class "6H" standard "ANSI Metric M Profile" full length
sketch "Sketch40" plane through (-17.3531, -3.7465, -46) normal (0, -1, 0) x (1, 0, 0)
  line L0 (0, 46.8535) -> (0, 0) projected
  line L1 (97.6, 46.8535) -> (97.6, 0) projected
  line L2 (20.8, 50) -> (76.8, 50)
  line L3 (76.8, 50) -> (76.8, -10)
  line L4 (76.8, -10) -> (20.8, -10)
  line L5 (20.8, -10) -> (20.8, 50)
  line L6 (48.8, 50) -> (48.8, 25.1181) construction
  line L7 (0, 2.6198) -> (97.6, 2.6198) construction
  line L8 (48.8, 2.6198) -> (48.8, 7.7623) construction
  line L9 (17.8, 57) -> (79.8, 57) construction
  point P0 (17.3531, 46)
  point P1 (39.5651, 57)
  point P2 (58.0349, 57)
  dimension "d270" = 56
  dimension "d272" = 60
  dimension "d273" = 7
  constraints: 14 end point, 3 parallel, 3 perpendicular, 2 midpoint, 2 point on line, 1 collinear, 1 horizontal
  measures "d270" distance of L2.start L2.end
  measures "d272" distance between parallel lines of L2 L4
  measures "d273" distance between parallel lines of L9 L2
extrude "Extrusion30" cut sketch "Sketch40" against normal blind 10
sketch "Sketch41" plane through (80.2469, -3.7465, -46) normal (0, -1, 0) x (1, 0, 0)
  line L0 (-76.8, 0) -> (-76.8, 50) projected
  line L1 (-20.8, 50) -> (-20.8, 0) projected
  line L2 (-80.3, 50) -> (-17.3, 50)
  line L3 (-17.3, 50) -> (-17.3, 53)
  line L4 (-17.3, 53) -> (-80.3, 53)
  line L5 (-80.3, 53) -> (-80.3, 50)
  point P0 (-80.2469, 46)
  dimension "d280" = 3.5
  dimension "d281" = 3.5
  dimension "d282" = 3
  dimension "d283" = 3
  constraints: 8 end point, 2 parallel, 1 horizontal, 1 perpendicular
  measures "d280" distance between parallel lines of L5 L0
  measures "d281" distance between parallel lines of L3 L1
  measures "d282" distance between parallel lines of L4 L2
  measures "d283" distance from line of L4 L1.start
extrude "Extrusion31" add sketch "Sketch41" against normal blind 2.5
body "Solid1"
